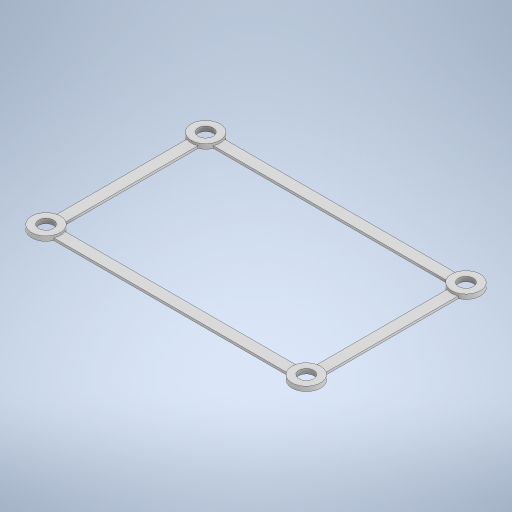
# Autodesk Inventor part: pcb_podstawka
Saved by Autodesk Inventor 2023.5 (Build 275446000, 446)
## iProperties
Created: 2025-03-16
Part Number: pcb_podstawka
Material: Ogólny
Document SubType Name: Modeling
Designer: kamil
Density: 1 g/cm^3
Appearance: Domyślna
Author: kamil
Autodesk Inventor part; units mm, degrees
ref_plane "YZ Plane" through (0, 0, 0) normal (1, 0, 0) x (0, 1, 0)
ref_plane "XZ Plane" through (0, 0, 0) normal (0, 1, 0) x (-1, 0, 0)
ref_plane "XY Plane" through (0, 0, 0) normal (0, 0, 1) x (1, 0, 0)
sketch "Szkic1" plane through (0, 0, 0) normal (0, 1, 0) x (-1, 0, 0)
  circle A0 centre (0, 0) radius 1.6
  circle A1 centre (0, -34.35) radius 1.6
  circle A2 centre (-56, 0) radius 1.6
  circle A3 centre (-56, -34.35) radius 1.6
  circle A4 centre (0, 0) radius 3.1
  circle A5 centre (-56, 0) radius 3.1
  circle A6 centre (0, -34.35) radius 3.1
  circle A7 centre (-56, -34.35) radius 3.1
  line L0 (0, 0) -> (0, -34.35)
  line L1 (0, -34.35) -> (-56, -34.35)
  line L2 (-56, -34.35) -> (-56, 0)
  line L3 (-56, 0) -> (0, 0)
  line L4 (1.2, -35.55) -> (1.2, 1.2)
  line L5 (1.2, 1.2) -> (-57.2, 1.2)
  line L6 (-57.2, 1.2) -> (-57.2, -35.55)
  line L7 (-57.2, -35.55) -> (1.2, -35.55)
  line L8 (-1.2, -33.15) -> (-1.2, -1.2)
  line L9 (-1.2, -1.2) -> (-54.8, -1.2)
  line L10 (-54.8, -1.2) -> (-54.8, -33.15)
  line L11 (-54.8, -33.15) -> (-1.2, -33.15)
  point P0 (1.2, -2.8583)
  point P1 (-2.8583, 1.2)
  point P2 (-53.1417, 1.2)
  point P3 (-57.2, -2.8583)
  point P4 (-57.2, -31.4917)
  point P5 (-53.1417, -35.55)
  point P6 (-2.8583, -35.55)
  point P7 (1.2, -31.4917)
  point P8 (-1.2, -2.8583)
  point P9 (-1.2, -31.4917)
  point P10 (-2.8583, -33.15)
  point P11 (-53.1417, -33.15)
  point P12 (-54.8, -31.4917)
  point P13 (-54.8, -2.8583)
  point P14 (-53.1417, -1.2)
  point P15 (-2.8583, -1.2)
  dimension "d0" = 56
  dimension "d1" = 34.35
  dimension "d2" = 3.2
  dimension "d3" = 3.2
  dimension "d4" = 3.2
  dimension "d5" = 3.2
  dimension "d6" = 1.5
  dimension "d7" = 1.5
  dimension "d8" = 1.5
  dimension "d9" = 1.5
  dimension "d10" = 1.2
  dimension "d11" = 1.2
  constraints: 24 end point, 9 perpendicular, 8 centre point, 5 coincident, 2 horizontal alignment, 2 vertical alignment, 1 vertical, 6 other
  measures "d0" distance of point (0, 0) point (-56, 0)
  measures "d1" distance of point (0, -34.35) point (0, 0)
  measures "d2" diameter of A0
  measures "d3" diameter of A1
  measures "d4" diameter of A2
  measures "d5" diameter of A3
  measures "d6" radial gap between concentric circles of A0 A4
  measures "d7" radial gap between concentric circles of A2 A5
  measures "d8" radial gap between concentric circles of A1 A6
  measures "d9" radial gap between concentric circles of A3 A7
  measures "d10" distance between parallel lines of L0 L4
  measures "d11" distance between parallel lines of L0 L8
extrude "Wyciągnięcie proste1" add sketch "Szkic1" along normal blind 0.5 contours A0 L4 | A0 L4 L5 A4 | L4 A0 L0 L3 L5 | A0 L5 L4 | L4 A4 L0 A0 | L5 A0 | L0 A4 L8 L9 L3 A0 | A0 L3 L0 | L4 A6 L0 A4 | A0 L3 A4 L5 | L0 A6 L8 A4 | L4 A1 L0 A6 | A6 L7 A1 L4 | A4 L3 A5 L5 | A4 L9 A5 L3 | A4 L9 L8 | L0 A1 L1 A6 L11 L8 | L4 A1 L7 L1 L0 | A1 L4 | L5 A2 L6 A5 | A5 L3 A2 L5 | A5 L9 L10 L2 A2 L3 | L8 L11 A6 | L0 L1 A1 | L7 A7 L1 A6 | A6 L1 A1 L7 | L4 L7 A1 | L6 A2 L2 A5 | A5 L2 A7 L6 | L5 A2 | A2 L3 L2 L6 L5 | A5 L10 L9 | A2 L2 L3 | A6 L1 A7 L11 | L7 A3 L1 A7 | A7 L6 A3 L7 | L7 A1 | A5 L10 A7 L2 | A2 L6 | A7 L2 A3 L6 | A2 L6 L5 | L11 L10 A7 | A7 L1 A3 L2 L10 L11 | L7 A3 L6 L2 L1 | A3 L7 | L6 A3 | L1 L2 A3 | L7 L6 A3
extrude "Wyciągnięcie proste2" add sketch "Szkic1" along normal blind 1 contours A0 L4 | A0 L4 L5 A4 | L4 A0 L0 L3 L5 | A0 L5 L4 | L4 A4 L0 A0 | L5 A0 | L0 A4 L8 L9 L3 A0 | A0 L3 L0 | A0 L3 A4 L5 | L4 A1 L0 A6 | A6 L7 A1 L4 | A4 L9 L8 | L0 A1 L1 A6 L11 L8 | L4 A1 L7 L1 L0 | A1 L4 | L5 A2 L6 A5 | A5 L3 A2 L5 | A5 L9 L10 L2 A2 L3 | L8 L11 A6 | L0 L1 A1 | A6 L1 A1 L7 | L4 L7 A1 | L6 A2 L2 A5 | L5 A2 | A2 L3 L2 L6 L5 | A5 L10 L9 | A2 L2 L3 | L7 A3 L1 A7 | A7 L6 A3 L7 | L7 A1 | A2 L6 | A7 L2 A3 L6 | A2 L6 L5 | L11 L10 A7 | A7 L1 A3 L2 L10 L11 | L7 A3 L6 L2 L1 | A3 L7 | L6 A3 | L1 L2 A3 | L7 L6 A3
sketch "Szkic2" plane through (0, 1, 0) normal (0, 1, 0) x (1, 0, 0)
  circle A0 centre (0, 0) radius 3.1 projected
  circle A1 centre (0, 34.35) radius 3.1 projected
  circle A2 centre (56, 0) radius 3.1 projected
  circle A3 centre (56, 34.35) radius 3.1 projected
hole "Otwór1" at (0, 1, 0) at (0, 1, -34.35) at (56, 1, -34.35) at (56, 1, 0) direction (0, -1, 0) diameter 3.2 depth 14 tip angle 118
